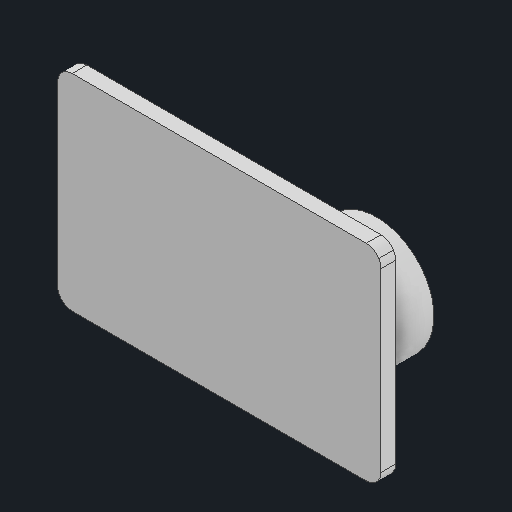
# Autodesk Inventor part: Top_part
Saved by Autodesk Inventor 2024.2 (Build 282272000, 272)
## iProperties
Created: 2024-03-21
Part Number: Top_part
Material: Generic
Document SubType Name: Modeling
Designer: seifs
Density: 1 g/cm^3
Appearance: Default
Author: seifs
Autodesk Inventor part; units mm, degrees
ref_plane "YZ Plane" through (0, 0, 0) normal (1, 0, 0) x (0, 1, 0)
ref_plane "XZ Plane" through (0, 0, 0) normal (0, 1, 0) x (-1, 0, 0)
ref_plane "XY Plane" through (0, 0, 0) normal (0, 0, 1) x (1, 0, 0)
sketch "Sketch1" plane through (0, 0, 0) normal (0, 0, 1) x (1, 0, 0)
  circle A0 centre (0, 0) radius 16.5 construction
  circle A1 centre (-46, 0.0011) radius 3 construction
  arc A2 (21.4991, -35.0005) -> (26.4993, -30.0007) centre (21.4993, -30.0005) ccw projected
  line L0 (26.4993, -30.0007) -> (26.5007, 29.9993) projected
  arc A3 (26.5007, 29.9993) -> (21.5009, 34.9995) centre (21.5007, 29.9995) ccw projected
  line L1 (21.5009, 34.9995) -> (-78.4991, 35.0019) projected
  arc A4 (-78.4991, 35.0019) -> (-83.4993, 30.0021) centre (-78.4993, 30.0019) ccw projected
  line L2 (-83.4993, 30.0021) -> (-83.5007, -29.9979) projected
  arc A5 (-83.5007, -29.9979) -> (-78.5009, -34.9981) centre (-78.5007, -29.9981) ccw projected
  line L3 (-78.5009, -34.9981) -> (21.4991, -35.0005) projected
  circle A6 centre (0, 0) radius 18.5 construction
  circle A7 centre (21.4993, -30.0005) radius 2.5 construction
  circle A8 centre (-78.5007, -29.9981) radius 2.5 construction
  circle A9 centre (21.5007, 29.9995) radius 2.5 construction
  circle A10 centre (-78.4993, 30.0019) radius 2.5 construction
  line L4 (-57.9994, 22.5014) -> (-67.4994, 22.5017) construction
  arc A11 (-67.4994, 22.5017) -> (-68.4995, 21.5017) centre (-67.4995, 21.5017) ccw construction
  line L5 (-68.4995, 21.5017) -> (-68.5005, -21.4983) construction
  arc A12 (-68.5005, -21.4983) -> (-67.5006, -22.4983) centre (-67.5005, -21.4983) ccw construction
  line L6 (-67.5006, -22.4983) -> (-24.5006, -22.4994) construction
  arc A13 (-24.5006, -22.4994) -> (-23.5005, -21.4994) centre (-24.5005, -21.4994) ccw construction
  line L7 (-23.4995, 21.5006) -> (-23.5005, -21.4994) construction
  arc A14 (-23.4995, 21.5006) -> (-24.4994, 22.5006) centre (-24.4995, 21.5006) ccw construction
  line L8 (-24.4994, 22.5006) -> (-33.9994, 22.5008) construction
  line L9 (-33.9994, 25.0008) -> (-33.9994, 22.5008) construction
  line L10 (-33.9994, 25.0008) -> (-22.9994, 25.0006) construction
  arc A15 (-20.9994, 23.0005) -> (-22.9994, 25.0006) centre (-22.9994, 23.0006) ccw construction
  line L11 (-20.9994, 23.0005) -> (-21.0006, -22.9995) construction
  arc A16 (-23.0006, -24.9994) -> (-21.0006, -22.9995) centre (-23.0006, -22.9994) ccw construction
  line L12 (-23.0006, -24.9994) -> (-69.0006, -24.9983) construction
  arc A17 (-71.0006, -22.9982) -> (-69.0006, -24.9983) centre (-69.0006, -22.9983) ccw construction
  line L13 (-71.0006, -22.9982) -> (-70.9994, 23.0018) construction
  arc A18 (-68.9994, 25.0017) -> (-70.9994, 23.0018) centre (-68.9994, 23.0017) ccw construction
  line L14 (-68.9994, 25.0017) -> (-57.9994, 25.0014) construction
  line L15 (-57.9994, 25.0014) -> (-57.9994, 22.5014) construction
  line L16 (21.4991, -35.0007) -> (-78.5007, -35.0007)
  line L17 (-83.5007, -30.0007) -> (-83.5007, 30.0021)
  line L18 (-78.5007, 35.0021) -> (21.4991, 35.0021)
  line L19 (26.4991, 30.0021) -> (26.4991, -30.0007)
  arc A19 (26.4991, 30.0021) -> (21.4991, 35.0021) centre (21.4991, 30.0021) ccw
  arc A20 (-78.5007, 35.0021) -> (-83.5007, 30.0021) centre (-78.5007, 30.0021) ccw
  arc A21 (-83.5007, -30.0007) -> (-78.5007, -35.0007) centre (-78.5007, -30.0007) ccw
  arc A22 (21.4991, -35.0007) -> (26.4991, -30.0007) centre (21.4991, -30.0007) ccw
  point P0 (0, 0)
  point P1 (26.4991, -35.0007)
  point P2 (-83.5007, 35.0021)
  point P3 (25.0347, -33.5362)
  point P4 (25.7513, 32.6325)
  dimension "d1" = 5
  constraints: 8 end point, 8 point on circle, 8 tangent, 6 point on line, 4 centre point, 3 equal radius, 2 parallel, 1 horizontal, 1 perpendicular
  measures "d1" radius of A19
extrude "Extrusion1" add sketch "Sketch1" along normal blind 5 contours L3 A5 L2 A4 L1 A3 L0 A2 | A3 L1 L18 A19
sketch "Sketch2" plane through (0, 0, 0) normal (0, 0, -1) x (-1, 0, 0)
  circle A0 centre (46, 0.0011) radius 3 construction
  circle A1 centre (0, 0) radius 16.5 projected
  circle A2 centre (0, 0) radius 16.5
  circle A3 centre (46, 0.0011) radius 11
  circle A4 centre (46, 0.0011) radius 14
  circle A5 centre (0, 0) radius 19.5
  point P0 (0, 0)
  dimension "d5" = 22
  dimension "d6" = 28
  dimension "d7" = 39
  constraints: 4 centre point, 4 coincident, 1 concentric
  measures "d5" diameter of A3
  measures "d6" diameter of A4
  measures "d7" diameter of A5
extrude "Extrusion2" add sketch "Sketch2" along normal blind 20
body "Solid1"
